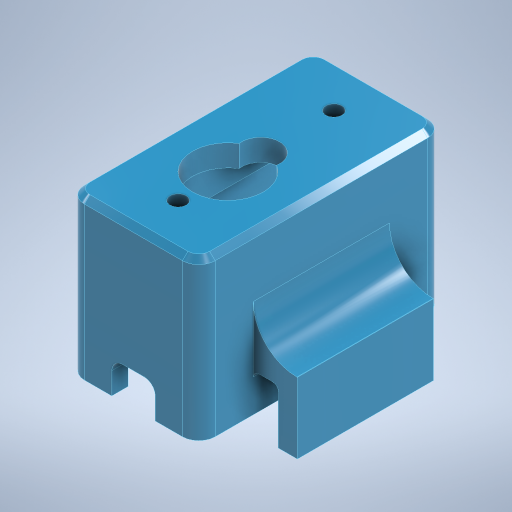
# Autodesk Inventor part: BaseRotativa
Saved by Autodesk Inventor 2024 (Build 280153000, 153)
## iProperties
Created: 2023-11-04
Part Number: BaseRotativa
Material: Generic
Document SubType Name: Modeling
Designer: fredy
Density: 1 g/cm^3
Appearance: Sky Blue Dark
Author: fredy
Autodesk Inventor part; units mm, degrees
ref_plane "YZ Plane" through (0, 0, 0) normal (1, 0, 0) x (0, 1, 0)
ref_plane "XZ Plane" through (0, 0, 0) normal (0, 1, 0) x (-1, 0, 0)
ref_plane "XY Plane" through (0, 0, 0) normal (0, 0, 1) x (1, 0, 0)
sketch "Sketch1" plane through (0, 0, 0) normal (0, 1, 0) x (-1, 0, 0)
  line L0 (12, 22.5) -> (-12, 22.5)
  line L1 (-12, 22.5) -> (-12, -22.5)
  line L2 (-12, -22.5) -> (12, -22.5)
  line L3 (12, -22.5) -> (12, 22.5)
  line L4 (12, 22.5) -> (-12, -22.5) construction
  line L5 (-12, 22.5) -> (12, -22.5) construction
  point P0 (0, 0)
  dimension "d20" = 45
  dimension "d21" = 24
  constraints: 12 end point, 2 midpoint, 2 parallel, 1 horizontal, 1 perpendicular
  measures "d20" distance of L0.end L1.end
  measures "d21" distance of L1.end L2.end
extrude "Extrusion1" add sketch "Sketch1" along normal blind 4
sketch "Sketch2" plane through (0, 4, 0) normal (0, 1, 0) x (1, 0, 0)
  line L0 (-16.8, 0) -> (16.8, 0) projected
  point P0 (0, 0)
  point P1 (0, 14.3)
  point P2 (0, -14.3)
  dimension "d8" = 28.6
  constraints: 1 symmetric about line, 1 vertical alignment
  measures "d8" distance of point (0, -14.3) point (0, 14.3)
hole "Hole1" at (0, 4, -14.3) at (0, 4, 14.3) direction (0, -1, 0) diameter 3 end through all
sketch "Sketch3" plane through (0, 4, 0) normal (0, 1, 0) x (1, 0, 0)
  line L0 (-6.5, -11.65) -> (6.5, -11.65)
  line L1 (6.5, -11.65) -> (6.5, 11.65)
  line L2 (6.5, 11.65) -> (-6.5, 11.65)
  line L3 (-6.5, 11.65) -> (-6.5, -11.65)
  line L4 (-6.5, -11.65) -> (6.5, 11.65) construction
  line L5 (6.5, -11.65) -> (-6.5, 11.65) construction
  circle A0 centre (0, -5.15) radius 6.5
  circle A1 centre (0, 0.85) radius 3.5
  circle A2 centre (0, -14.3) radius 1.5 projected
  point P0 (0, 0)
  point P1 (-3.4641, 0.35)
  point P2 (-4.6637, -11.65)
  point P3 (0, -11.65)
  point P4 (3.4641, 0.35)
  dimension "d16" = 13
  dimension "d17" = 23.3
  dimension "d38" = 13
  dimension "d39" = 7
  dimension "d40" = 6
  dimension "d41" = 9.15
  constraints: 12 end point, 2 centre point, 2 midpoint, 2 parallel, 2 vertical alignment, 1 horizontal, 1 perpendicular
  measures "d16" distance of L0.start L0.end
  measures "d17" distance of L0.end L1.end
  measures "d38" diameter of A0
  measures "d39" diameter of A1
  measures "d40" distance of A0.centre A1.centre
  measures "d41" distance of A2.centre A0.centre
extrude "Extrusion2" cut sketch "Sketch3" against normal up to surface (4 mm away) contours A0 A1 | A1 A0 | A0 A1
fillet "Fillet1" radius 3 4 edges at (-12, 2, -22.5) (-12, 2, 22.5) (12, 2, 22.5) (12, 2, -22.5)
sketch "Sketch4" plane through (0, 0, 0) normal (0, -1, 0) x (1, 0, 0)
  line L0 (-9, 22.5) -> (9, 22.5) projected
  arc A0 (-9, 22.5) -> (-12, 19.5) centre (-9, 19.5) ccw projected
  line L1 (-12, -19.5) -> (-12, 19.5) projected
  arc A1 (-12, -19.5) -> (-9, -22.5) centre (-9, -19.5) ccw projected
  line L2 (9, -22.5) -> (-9, -22.5) projected
  arc A2 (9, -22.5) -> (12, -19.5) centre (9, -19.5) ccw projected
  line L3 (12, 19.5) -> (12, -19.5) projected
  arc A3 (12, 19.5) -> (9, 22.5) centre (9, 19.5) ccw projected
  line L4 (-9, 17.5) -> (-9, -17.5)
  line L5 (-7, -19.5) -> (7, -19.5)
  line L6 (9, -17.5) -> (9, 17.5)
  line L7 (7, 19.5) -> (-7, 19.5)
  arc A4 (-7, 19.5) -> (-9, 17.5) centre (-7, 17.5) ccw
  arc A5 (-9, -17.5) -> (-7, -19.5) centre (-7, -17.5) ccw
  arc A6 (7, -19.5) -> (9, -17.5) centre (7, -17.5) ccw
  arc A7 (9, 17.5) -> (7, 19.5) centre (7, 17.5) ccw
  point P0 (0, 0)
  dimension "d23" = 2
  dimension "d24" = 3
  dimension "d25" = 3
  dimension "d26" = 3
  dimension "d27" = 3
  constraints: 8 end point, 8 point on circle, 8 tangent, 4 centre point, 3 equal radius, 1 horizontal, 1 parallel, 1 perpendicular, 1 vertical
  measures "d23" radius of A4
  measures "d24" distance between parallel lines of L7 L0
  measures "d25" distance between parallel lines of L1 L4
  measures "d26" distance between parallel lines of L2 L5
  measures "d27" distance between parallel lines of L3 L6
extrude "Extrusion3" add sketch "Sketch4" along normal blind 25
chamfer "Chamfer1" distance 1 angle 45 8 edges at (-12, 4, 0) (-11.1213, 4, 21.6213) (0, 4, 22.5) (11.1213, 4, 21.6213) (12, 4, 0) (11.1213, 4, -21.6213) (0, 4, -22.5) (-11.1213, 4, -21.6213)
sketch "Sketch5" plane through (-9, -25, 22.5) normal (0, 0, 1) x (1, 0, 0)
  line L0 (5, 0) -> (13, 0)
  line L1 (13, 0) -> (13, 6)
  line L2 (13, 6) -> (5, 6)
  line L3 (5, 6) -> (5, 0)
  line L4 (18, 0) -> (0, 0) projected
  point P0 (9, 25)
  point P1 (9, 6)
  dimension "d33" = 8
  dimension "d34" = 6
  constraints: 8 end point, 2 parallel, 1 horizontal, 1 midpoint, 1 perpendicular, 1 point on line, 1 vertical alignment
  measures "d33" distance of L1.end L2.end
  measures "d34" distance of L0.end L1.end
extrude "Extrusion4" cut sketch "Sketch5" against normal up to surface (3 mm away)
fillet "Fillet2" radius 2 2 edges at (-4, -19, 21) (4, -19, 21)
sketch "Sketch6" plane through (0, 0, 0) normal (0, -1, 0) x (1, 0, 0)
  line L0 (9, 17.5) -> (9, -17.5) projected
  arc A0 (9, 17.5) -> (7, 19.5) centre (7, 17.5) ccw projected
  line L1 (7, 19.5) -> (-7, 19.5) projected
  arc A1 (-7, 19.5) -> (-9, 17.5) centre (-7, 17.5) ccw projected
  line L2 (-9, 17.5) -> (-9, -17.5) projected
  arc A2 (-9, -17.5) -> (-7, -19.5) centre (-7, -17.5) ccw projected
  line L3 (-7, -19.5) -> (7, -19.5) projected
  arc A3 (7, -19.5) -> (9, -17.5) centre (7, -17.5) ccw projected
  circle A4 centre (0, 14.3) radius 1.5 projected
  circle A5 centre (0, -14.3) radius 1.5 projected
  arc A6 (3.4641, -0.35) -> (-3.4641, -0.35) centre (0, 5.15) ccw projected
  arc A7 (-3.4641, -0.35) -> (3.4641, -0.35) centre (0, -0.85) ccw projected
  line L4 (-6.5, 12) -> (6.5, 12)
  line L5 (6.5, 12) -> (6.5, -12)
  line L6 (6.5, -12) -> (-6.5, -12)
  line L7 (-6.5, -12) -> (-6.5, 12)
  line L8 (-6.5, 12) -> (6.5, -12) construction
  line L9 (6.5, 12) -> (-6.5, -12) construction
  point P0 (0, 0)
  dimension "d44" = 13
  dimension "d45" = 24
  constraints: 12 end point, 2 midpoint, 2 parallel, 1 horizontal, 1 perpendicular
  measures "d44" distance of L5.end L6.end
  measures "d45" distance of L4.end L5.end
extrude "Extrusion5" add sketch "Sketch6" along normal blind 5
sketch "Sketch7" plane through (0, 0, 0) normal (0, 0, 1) x (1, 0, 0)
  line L0 (-12, 3) -> (-12, -25) projected
  line L1 (-12, -15) -> (-20.1, -15)
  line L2 (-20.1, -15) -> (-20.1, -28)
  line L3 (-20.1, -28) -> (-16.6, -28)
  line L4 (-16.6, -28) -> (-16.6, -18)
  line L5 (-16.6, -18) -> (-12, -18)
  line L6 (-12, -15) -> (-12, -18)
  line L7 (0, 9.2) -> (0, -34.2) projected
  line L8 (12, -15) -> (20.1, -15)
  line L9 (20.1, -15) -> (20.1, -28)
  line L10 (20.1, -28) -> (16.6, -28)
  line L11 (16.6, -28) -> (16.6, -18)
  line L12 (16.6, -18) -> (12, -18)
  line L13 (12, -15) -> (12, -18)
  point P0 (0, 0)
  point P1 (-14.3, -18)
  point P2 (12, -25)
  point P3 (14.3, -18)
  dimension "d47" = 4.6
  dimension "d48" = 3.5
  dimension "d49" = 7
  dimension "d50" = 3
  dimension "d52" = 10
  constraints: 24 end point, 8 symmetric about line, 4 perpendicular, 2 point on line, 1 collinear, 1 midpoint, 1 vertical
  measures "d47" horizontal distance of L3.end L5.end
  measures "d48" distance of L3.end L2.end
  measures "d49" distance from line of L5 L0.end
  measures "d50" distance from line of point (-14.3, -18) L1
  measures "d52" vertical distance of L2.end point (-14.3, -18)
extrude "Extrusion6" add sketch "Sketch7" along normal mid plane 25
fillet "Fillet3" radius 8 2 edges at (-12, -15, 0) (12, -15, 0)
fillet "Fillet4" radius 1 4 edges at (-16.6, -18, 0) (16.6, -18, 0) (-12, -18, 0) (12, -18, 0)
body "Solid1"
